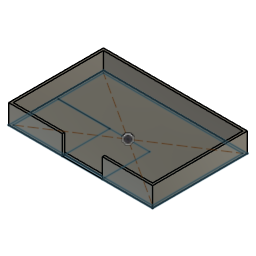
RPI_display_holder_5in (Autodesk Fusion 360 design; units mm, degrees)
part number: 2025-07-09-18-37-19-838
part number: 2025-07-09-18-37-26-636
Autodesk Fusion 360 part; units mm, degrees
sketch "Sketch1" plane through (0, 0, 0) normal (0, 0, 1) x (1, 0, 0) in component "stand"
  line L0 (61, -39.5) -> (-61, -39.5)
  line L1 (-61, -39.5) -> (-61, 39.5)
  line L2 (-61, 39.5) -> (61, 39.5)
  line L3 (61, 39.5) -> (61, -39.5)
  line L4 (61, -39.5) -> (-61, 39.5) construction
  line L5 (-61, -39.5) -> (61, 39.5) construction
  line L6 (63, -41.5) -> (-63, -41.5)
  line L7 (-63, -41.5) -> (-63, 41.5)
  line L8 (-63, 41.5) -> (63, 41.5)
  line L9 (63, 41.5) -> (63, -41.5)
  line L10 (-61, 0) -> (-16, 0)
  line L11 (-61, 0) -> (19, 0)
  line L12 (-16, 0) -> (-16, -41.5)
  line L13 (19, 0) -> (19, -41.5)
  line L14 (-61, 39.5) -> (61, 39.5)
  line L15 (-61, 0) -> (19, 0)
  line L16 (-63, 41.5) -> (63, 41.5)
  line L17 (-63, -41.5) -> (-63, 41.5)
  line L18 (-61, 0) -> (-16, 0)
  line L19 (63, 41.5) -> (63, -41.5)
  line L20 (61, 39.5) -> (61, -39.5)
  line L21 (-16, 0) -> (-16, -41.5)
  line L22 (61, -39.5) -> (-61, -39.5)
  line L23 (63, -41.5) -> (-63, -41.5)
  line L24 (-61, -39.5) -> (-61, 39.5)
  line L25 (61, -39.5) -> (-61, 39.5) construction
  line L26 (19, 0) -> (19, -41.5)
  line L27 (-61, -39.5) -> (61, 39.5) construction
  dimension "d1" = 122
  dimension "d2" = 79
  dimension "d3" = -2
  dimension "d4" = 45
  dimension "d5" = 80
  dimension "d10" = -2
  dimension "d11" = 122
  dimension "d12" = 79
  dimension "d13" = 45
  dimension "d14" = 80
  constraint horizontal L0
  constraint perpendicular L0 L1
  constraint parallel L0 L2
  constraint parallel L1 L3
  constraint coincident L4 origin
  constraint coincident L5 origin
  constraint midpoint L1 L10.start
  constraint perpendicular L1 L10
  constraint parallel L10 L11
  constraint coincident L6 L12.end
  constraint perpendicular L6 L12
  constraint coincident L6 L13.end
  constraint perpendicular L6 L13
  constraint horizontal L22
  constraint perpendicular L22 L24
  constraint parallel L14 L22
  constraint parallel L20 L24
  constraint coincident origin L25
  constraint coincident origin L27
  constraint midpoint L10.start L24
  constraint perpendicular L18 L24
  constraint parallel L15 L18
  constraint coincident L12.end L23
  constraint perpendicular L21 L23
  constraint coincident L13.end L23
  constraint perpendicular L23 L26
  measures "d1" distance of L1.end L2.end
  measures "d2" distance of L0.end L1.end
  measures "d4" distance of L10.start L10.end
  measures "d5" distance of L10.start L11.end
  measures "d11" distance of L2.end L1.end
  measures "d12" distance of L0.end L1.end
  measures "d13" distance of L10.end L10.start
  measures "d14" distance of L11.end L10.start
extrude "Extrude1" add sketch "Sketch1" along normal blind 17 contours L0 L1 L2 L3 L6 L7 L8 L9 L12 L13 L14 L16 L17 L19 L20 L21 L22 L23 L24 L26 in component "stand"
extrude "Extrude2" add sketch "Sketch1" along normal blind 2 contours L0 L1 L2 L3 L10 L11 L13 L14 L15 L18 L20 L22 L24 L26 | L0 L11 L12 L13 L15 L21 L22 L26 | L0 L1 L10 L11 L12 L15 L18 L21 L22 L24 in component "stand"
component "stand" placed x (1, 0, 0) y (0, 1, 0) z (0, 0, 1) at (0, 0, 0)
